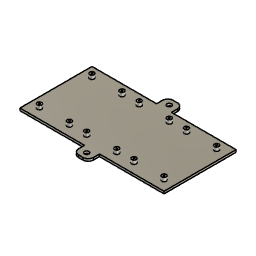
wt_shelf_mount_1 v1 (Autodesk Fusion 360 design; units mm, degrees)
Autodesk Fusion 360 part; units mm, degrees
sketch "Sketch1" plane through (0, 0, 0) normal (0, 0, 1) x (1, 0, 0)
  line L0 (0, 0) -> (192, 0)
  line L1 (192, 0) -> (192, 96)
  line L2 (192, 96) -> (0, 96)
  line L3 (0, 96) -> (0, 0)
  dimension "d1" = 192
  dimension "d2" = 96
  constraint horizontal L0
  constraint vertical L1
  constraint horizontal L2
  constraint vertical L3
  constraint coincident L0.start L3.end
  measures "d1" distance of L0.start L0.end
  measures "d2" distance of L0.start L2.end
extrude "Extrude1" add sketch "Sketch1" along normal blind 3
sketch "Sketch3" plane through (0, 0, 3) normal (0, 0, 1) x (-1, 0, 0)
  line L0 (0, -96) -> (0, 0)
  line L1 (0, 0) -> (-192, 0)
  line L2 (-192, 0) -> (-192, -96)
  line L3 (-192, -96) -> (0, -96)
  line L4 (-3, -93) -> (-63, -93)
  line L5 (-63, -93) -> (-63, -3)
  line L6 (-63, -3) -> (-3, -3)
  line L7 (-3, -3) -> (-3, -93)
  circle A0 centre (-13, -83) radius 1
  circle A1 centre (-53, -83) radius 1
  circle A2 centre (-13, -13) radius 1
  circle A3 centre (-53, -13) radius 1
  circle A4 centre (-13, -83) radius 3
  circle A5 centre (-53, -83) radius 3
  circle A6 centre (-13, -13) radius 3
  circle A7 centre (-53, -13) radius 3
  dimension "d7" = 60
  dimension "d8" = 90
  dimension "d9" = 3
  dimension "d10" = 3
  dimension "d11" = 2
  dimension "d12" = 10
  dimension "d13" = 10
  dimension "d14" = 2
  dimension "d15" = 10
  dimension "d16" = 10
  dimension "d17" = 2
  dimension "d18" = 10
  dimension "d19" = 10
  dimension "d20" = 2
  dimension "d21" = 10
  dimension "d22" = 10
  dimension "d23" = 6
  dimension "d24" = 6
  dimension "d25" = 6
  dimension "d26" = 6
  constraint horizontal L4
  constraint vertical L5
  constraint horizontal L6
  constraint vertical L7
  constraint concentric A0 A4
  constraint concentric A1 A5
  constraint concentric A2 A6
  constraint concentric A3 A7
  measures "d7" distance of L4.start L4.end
  measures "d8" distance of L4.start L6.end
  measures "d9" distance of L3 L4
  measures "d10" distance of L0 L7
  measures "d11" diameter of A0
  measures "d12" distance of L7 A0.centre
  measures "d13" distance of L4 A0.centre
  measures "d14" diameter of A1
  measures "d15" distance of L5 A1.centre
  measures "d16" distance of L4 A1.centre
  measures "d17" diameter of A2
  measures "d18" distance of L6 A2.centre
  measures "d19" distance of L7 A2.centre
  measures "d20" diameter of A3
  measures "d21" distance of L5 A3.centre
  measures "d22" distance of L6 A3.centre
  measures "d23" diameter of A4
  measures "d24" diameter of A5
  measures "d25" diameter of A6
  measures "d26" diameter of A7
extrude "Extrude2" add sketch "Sketch3" along normal blind 5 contours A4 | A5 | A6 | A7
sketch "Sketch4" plane through (0, 0, 3) normal (0, 0, 1) x (-1, 0, 0)
  circle A0 centre (-13, -83) radius 3
  circle A1 centre (-53, -83) radius 3
  line L0 (0, -96) -> (0, 0)
  line L1 (0, 0) -> (-192, 0)
  line L2 (-192, 0) -> (-192, -96)
  line L3 (-192, -96) -> (0, -96)
  circle A2 centre (-53, -13) radius 3
  circle A3 centre (-13, -13) radius 3
  line L4 (-66, -3) -> (-66, -93)
  circle A4 centre (-116, -13) radius 3
  line L5 (-66, -93) -> (-126, -93)
  line L6 (-126, -3) -> (-66, -3)
  circle A5 centre (-76, -13) radius 3
  circle A6 centre (-76, -83) radius 3
  line L7 (-126, -93) -> (-126, -3)
  circle A7 centre (-76, -13) radius 1
  circle A8 centre (-116, -83) radius 3
  circle A9 centre (-116, -13) radius 1
  line L8 (-63, -96) -> (-63, 0)
  circle A10 centre (-116, -83) radius 1
  circle A11 centre (-76, -83) radius 1
  line L9 (-129, -3) -> (-129, -93)
  circle A12 centre (-179, -13) radius 3
  line L10 (-129, -93) -> (-189, -93)
  line L11 (-189, -3) -> (-129, -3)
  circle A13 centre (-139, -13) radius 3
  circle A14 centre (-139, -83) radius 3
  line L12 (-189, -93) -> (-189, -3)
  circle A15 centre (-139, -13) radius 1
  circle A16 centre (-179, -83) radius 3
  circle A17 centre (-179, -13) radius 1
  line L13 (-126, -96) -> (-126, 0)
  circle A18 centre (-179, -83) radius 1
  circle A19 centre (-139, -83) radius 1
  point P0 (-63, 0)
  point P1 (-126, 0)
  dimension "d29" = 60
  dimension "d30" = 90
  dimension "d31" = 3
  dimension "d32" = 2
  dimension "d33" = 10
  dimension "d34" = 10
  dimension "d35" = 2
  dimension "d36" = 10
  dimension "d37" = 10
  dimension "d38" = 2
  dimension "d39" = 10
  dimension "d40" = 10
  dimension "d41" = 2
  dimension "d42" = 10
  dimension "d43" = 10
  dimension "d44" = 6
  dimension "d45" = 6
  dimension "d46" = 6
  dimension "d47" = 6
  dimension "d48" = 60
  dimension "d49" = 90
  dimension "d50" = 3
  dimension "d51" = 2
  dimension "d52" = 10
  dimension "d53" = 10
  dimension "d54" = 2
  dimension "d55" = 10
  dimension "d56" = 10
  dimension "d57" = 2
  dimension "d58" = 10
  dimension "d59" = 10
  dimension "d60" = 2
  dimension "d61" = 10
  dimension "d62" = 10
  dimension "d63" = 6
  dimension "d64" = 6
  dimension "d65" = 6
  dimension "d66" = 6
  constraint horizontal L5
  constraint vertical L7
  constraint horizontal L6
  constraint vertical L4
  constraint concentric A6 A11
  constraint concentric A8 A10
  constraint concentric A5 A7
  constraint concentric A4 A9
  constraint horizontal L10
  constraint vertical L12
  constraint horizontal L11
  constraint vertical L9
  constraint concentric A14 A19
  constraint concentric A16 A18
  constraint concentric A13 A15
  constraint concentric A12 A17
  measures "d29" distance of L5.end L4.end
  measures "d30" distance of L4.start L4.end
  measures "d31" distance of L4 L8
  measures "d32" diameter of A11
  measures "d33" distance of A6.centre L4
  measures "d34" distance of A6.centre L5
  measures "d35" diameter of A10
  measures "d36" distance of A8.centre L7
  measures "d37" distance of A8.centre L5
  measures "d38" diameter of A7
  measures "d39" distance of A5.centre L6
  measures "d40" distance of A5.centre L4
  measures "d41" diameter of A9
  measures "d42" distance of A4.centre L7
  measures "d43" distance of A4.centre L6
  measures "d44" diameter of A6
  measures "d45" diameter of A8
  measures "d46" diameter of A5
  measures "d47" diameter of A4
  measures "d48" distance of L10.end L9.end
  measures "d49" distance of L9.start L9.end
  measures "d50" distance of L9 L13
  measures "d51" diameter of A19
  measures "d52" distance of A14.centre L9
  measures "d53" distance of A14.centre L10
  measures "d54" diameter of A18
  measures "d55" distance of A16.centre L12
  measures "d56" distance of A16.centre L10
  measures "d57" diameter of A15
  measures "d58" distance of A13.centre L11
  measures "d59" distance of A13.centre L9
  measures "d60" diameter of A17
  measures "d61" distance of A12.centre L12
  measures "d62" distance of A12.centre L11
  measures "d63" diameter of A14
  measures "d64" diameter of A16
  measures "d65" diameter of A13
  measures "d66" diameter of A12
extrude "Extrude3" add sketch "Sketch4" along normal blind 5 contours A4 | A5 | A6 | A8 | A12 | A13 | A14 | A16
sketch "Sketch5" plane through (0, 0, 3) normal (0, 0, 1) x (-1, 0, 0)
  circle A0 centre (-179, -83) radius 3
  circle A1 centre (-179, -13) radius 3
  circle A2 centre (-139, -83) radius 3
  circle A3 centre (-139, -13) radius 3
  circle A4 centre (-13, -83) radius 3
  circle A5 centre (-53, -83) radius 3
  line L0 (0, -96) -> (0, 0)
  line L1 (0, 0) -> (-192, 0)
  line L2 (-192, 0) -> (-192, -96)
  line L3 (-192, -96) -> (0, -96)
  circle A6 centre (-53, -13) radius 3
  circle A7 centre (-13, -13) radius 3
  circle A8 centre (-116, -83) radius 3
  circle A9 centre (-116, -13) radius 3
  circle A10 centre (-76, -83) radius 3
  circle A11 centre (-76, -13) radius 3
  line L4 (-86, -96) -> (-106, -96)
  line L5 (-106, -96) -> (-106, -104)
  line L6 (-99, -111) -> (-93, -111)
  line L7 (-86, -104) -> (-86, -96)
  circle A12 centre (-96, -103) radius 3
  arc A13 (-93, -111) -> (-86, -104) centre (-93, -104) ccw
  arc A14 (-106, -104) -> (-99, -111) centre (-99, -104) ccw
  line L8 (0, -48) -> (-192, -48)
  arc A15 (-86, 8) -> (-93, 15) centre (-93, 8) ccw
  arc A16 (-99, 15) -> (-106, 8) centre (-99, 8) ccw
  line L9 (-86, 0) -> (-106, 0)
  line L10 (-86, 8) -> (-86, 0)
  line L11 (-106, 0) -> (-106, 8)
  circle A17 centre (-96, 7) radius 3
  line L12 (-99, 15) -> (-93, 15)
  line L13 (-192, 0) -> (0, 0)
  point P0 (-86, -111)
  point P1 (-86, 15)
  dimension "d69" = 20
  dimension "d70" = 15
  dimension "d71" = 6
  dimension "d72" = 7
  dimension "d73" = 7
  constraint horizontal L4
  constraint vertical L5
  constraint horizontal L6
  constraint vertical L7
  constraint coincident L3 L4.start
  constraint midpoint L3 L4
  constraint coincident P0 L6
  constraint coincident P0 L7
  constraint tangent L6 A13
  constraint tangent L7 A13
  constraint tangent L5 A14
  constraint tangent L6 A14
  constraint equal A13 A14
  constraint midpoint L0 L8.start
  constraint midpoint L2 L8.end
  constraint symmetric L0.start L8 L0.end
  constraint symmetric L2.end L8 L1.end
  constraint symmetric L4.start L8 L9.start
  constraint symmetric L4.end L8 L9.end
  constraint symmetric P0 L8 P1
  constraint symmetric A12 L8 A17
  constraint symmetric L6.end L8 A15.end
  constraint symmetric L7.start L8 A15.start
  constraint symmetric A13 L8 A15
  constraint symmetric L5.end L8 A16.end
  constraint symmetric L6.start L8 A16.start
  constraint symmetric A14 L8 A16
  measures "d69" distance of L4.start L4.end
  measures "d70" distance of L4.start P0
  measures "d71" diameter of A12
  measures "d72" distance of L4 A12.centre
  measures "d73" radius of A13
extrude "Extrude4" add sketch "Sketch5" against normal blind 3 contours L3 L4 L5 L6 L7 A13 A14 | L1 A15 A16 L9 L10 L11 L12 L13
